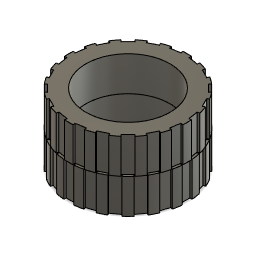
MacrobotSketch (Autodesk Fusion 360 archive; units mm, degrees)
design "Tire (1)"
Autodesk Fusion 360 part; units mm, degrees
cylinder "CylinderPrimitive1" add diameter 24 height 14 placed x (1, 0, 0) y (0, 0, -1) z (0, 1, 0) at (0, 0, 0) makes body 1
sketch "Sketch2" plane through (0, 14, 0) normal (0, 1, 0) x (-1, 0, 0)
  circle A0 centre (0, 0) radius 12
  circle A1 centre (0, 0) radius 8.5
  dimension "d3" = -3.5
extrude "Extrude1" cut sketch "Sketch2" against normal blind 44 contours A1 bodies 1
box "BoxPrimitive1" add length 2 width 2 height 2 placed x (0, 0, -1) y (-1, 0, 0) z (0, 1, 0) at (2, 0, 0) separate body makes body 2
move_body "Move1" bodies 2 to x (1, 0, 0) y (0, 1, 0) z (0, 0, 1) at (11, 0, 1)
extrude "Extrude2" cut 1 faces at (10.757, 14, 1.0185) along direction (0, -1, 0) blind 7 on bodies 1 bodies 1
extrude "Extrude3" add 1 faces at (11.6667, 2, 0.3333) along direction (0, 1, 0) blind 14 on bodies 2 bodies 2
move_body "Move2" bodies 2 to x (1, 0, 0) y (0, 1, 0) z (0, 0, 1) at (0, -2.5, 0)
move_body "Move3" bodies 2 to x (1, 0, 0) y (0, 1, 0) z (0, 0, 1) at (0.5, 0, 0)
pattern_circular "C-Pattern1" count 20 over 360 about axis through (0, 1.75, 0) along (0, 1, 0) of bodies 2 makes body 3 at (11.8802, 2.8333, -2.8087) makes body 4 at (10.4308, 2.8333, -6.3424) makes body 5 at (7.9604, 2.8333, -9.2553) makes body 6 at (4.9168, 8.1667, -11.8962) makes body 7 at (1, 2.8333, -12.1667) makes body 8 at (-2.8087, 2.8333, -11.8802) makes body 9 at (-6.3424, 2.8333, -10.4308) makes body 10 at (-9.2553, 2.8333, -7.9604) makes body 11 at (-11.2622, 2.8333, -4.7108) makes body 12 at (-12.1667, 2.8333, -1) makes body 13 at (-11.8802, 2.8333, 2.8087) makes body 14 at (-10.4308, 2.8333, 6.3424) makes body 15 at (-7.9604, 2.8333, 9.2553) makes body 16 at (-4.9168, 8.1667, 11.8962) makes body 17 at (-1, 2.8333, 12.1667) makes body 18 at (2.8087, 2.8333, 11.8802) makes body 19 at (6.7342, 8.1667, 10.9702) makes body 20 at (9.2553, 2.8333, 7.9604) makes body 21 at (11.2622, 2.8333, 4.7108)
combine "Combine1" operation cut target body 1 tool bodies 2 8 6 21 5 4 3 7 18 19 16 15 17 20 12 14 13 11 9 10
copy_body "CopyPasteBodies1" bodies 1 makes body 22
move_body "Move4" bodies 22 to x (1, 0, 0) y (0, 1, 0) z (0, 0, 1) at (0, 7, 0)
move_body "Move5" bodies 22 to x (0.987688, 0, -0.156434) y (0, 1, 0) z (0.156434, 0, 0.987688) at (0, 0, 0)
